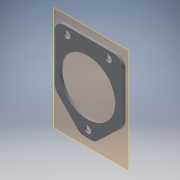
# Autodesk Inventor part: 30_Cube_Insert_Filter_Revolver_Filter_clamp_v3
Saved by Autodesk Inventor 2019.4 (Build 234330000, 330)
## iProperties
Created: 2021-09-14
Part Number: 30_Cube_Insert_Filter_Revolver_Filter_clamp_v3
Material: Generic
Document SubType Name: Modeling
Designer: diederichbenedict
Density: 1 g/cm^3
Appearance: Default
Mass: 0.70962 g
Surface Area: 14.1923 cm^2
Volume: 0.70962 cm^3
Author: diederichbenedict
Autodesk Inventor part; units mm, degrees
ref_plane "YZ Plane" through (0, 0, 0) normal (1, 0, 0) x (0, 1, 0)
ref_plane "XZ Plane" through (0, 0, 0) normal (0, 1, 0) x (-1, 0, 0)
ref_plane "XY Plane" through (0, 0, 0) normal (0, 0, 1) x (1, 0, 0)
ref_plane "Work Plane1" through (1.8898, -14.3412, -20.7656) normal (0, 0, 1) x (1, 0, 0)
sketch "Sketch5" plane through (1.8898, -14.3412, -20.7656) normal (0, 0, 1) x (1, 0, 0)
  circle A0 centre (-14.5, 20.385) radius 12.5 projected
  circle A1 centre (-6, 34.885) radius 1.45 projected
  circle A2 centre (-14.5, 5.385) radius 1.45 projected
  circle A3 centre (-23, 34.885) radius 1.45 projected
  ellipse E0 centre (-14.5, 20.385) end of major axis (-14.5, 38.4869) minor radius 12.8 (-11.7974, 38.0788) -> (-17.2026, 38.0788) ccw projected
  line L0 (-11.7974, 38.0788) -> (-17.2026, 38.0788) projected
  circle A4 centre (-14.5, 20.385) radius 12.75 projected
  ellipse E1 centre (-39.78, 51.5138) end of major axis (-39.78, -18.2605) minor radius 49.3379 (-6.5026, 0) -> (0, 10.2397) ccw projected
  line L1 (0, 10.2397) -> (0, 38.9273) projected
  line L2 (0, 38.9273) -> (-28, 38.9273) projected
  line L3 (-28, 0) -> (-28, 38.9273) projected
  line L4 (-6.5026, 0) -> (-28, 0) projected
  circle A5 centre (-14.5, 20.385) radius 11.3498
  line L5 (-11.5, 2.385) -> (-17.5, 2.385)
  line L6 (-17.5, 2.385) -> (-28, 13.3623)
  line L7 (0, 37.885) -> (-28, 37.885)
  line L8 (-28, 13.3623) -> (-28, 37.885)
  line L9 (0, 37.885) -> (0, 13.385)
  line L10 (-11.5, 2.385) -> (0, 13.385)
  point P0 (-1.8898, 14.3412)
  dimension "d34" = 3
  dimension "d35" = 3
  dimension "d36" = 3
  dimension "d37" = 8
  dimension "d38" = 3
  constraints: 12 end point, 4 point on line, 2 perpendicular, 1 centre point, 1 collinear, 1 horizontal, 2 other
  measures "d34" distance from line of L5 A2.centre
  measures "d35" horizontal distance of L5.end A2.centre
  measures "d36" horizontal distance of L5.start A2.centre
  measures "d37" vertical distance of L9.end A2.centre
  measures "d38" distance from line of L7 A1.centre
extrude "Extrusion5" add sketch "Sketch5" along normal blind 1 contours A0 | A4 | L10 L5 L6 L3 L7 L1
fillet "Fillet3" radius 4 6 edges at (-26.1102, -0.979, -20.2656) (-15.6102, -11.9562, -20.2656) (-9.6102, -11.9562, -20.2656) (1.8898, -0.9562, -20.2656) (1.8898, 23.5438, -20.2656) (-26.1102, 23.5438, -20.2656)
body "Solid2"
